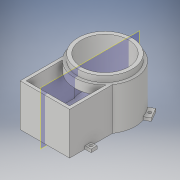
# Autodesk Inventor part: table
Saved by Autodesk Inventor 2018 (Build 220112000, 112)
## iProperties
Created: 2018-04-17
Part Number: table
Material: Generic
Document SubType Name: Modeling
Designer: Cole Tucker
Density: 1 g/cm^3
Appearance: Default
Author: Cole Tucker
Autodesk Inventor part; units mm, degrees
ref_plane "YZ Plane" through (0, 0, 0) normal (1, 0, 0) x (0, 1, 0)
ref_plane "XZ Plane" through (0, 0, 0) normal (0, 1, 0) x (-1, 0, 0)
ref_plane "XY Plane" through (0, 0, 0) normal (0, 0, 1) x (1, 0, 0)
sketch "Sketch1" plane through (0, 0, 0) normal (0, 1, 0) x (-1, 0, 0)
  circle A0 centre (0, 0) radius 24.765
  circle A1 centre (0, 0) radius 28.575
  dimension "d0" = 49.53
  dimension "d1" = 57.15
  constraints: 2 centre point, 2 coincident
  measures "d0" diameter of A0
  measures "d1" diameter of A1
extrude "Extrusion1" add sketch "Sketch1" along normal blind 50.8
sketch "Sketch2" plane through (0, 0, 0) normal (0, -1, 0) x (1, 0, 0)
  circle A0 centre (0, 0) radius 31.75
  circle A1 centre (0, 0) radius 24.765 projected
  circle A2 centre (0, 0) radius 28.575 projected
  circle A3 centre (0, 0) radius 28.575
  dimension "d4" = 63.5
  constraints: 2 centre point, 2 coincident
  measures "d4" diameter of A0
extrude "Extrusion2" add sketch "Sketch2" against normal blind 44.45 contours A0
sketch "Sketch3" plane through (0, 0, 0) normal (0, -1, 0) x (1, 0, 0)
  circle A0 centre (0, 0) radius 24.765 projected
  line L0 (0, 24.765) -> (6.35, 24.765)
  line L1 (6.35, 24.765) -> (6.35, 37.465)
  line L2 (6.35, 37.465) -> (-6.35, 37.465)
  line L3 (-6.35, 37.465) -> (-6.35, 24.765)
  line L4 (-6.35, 24.765) -> (0, 24.765)
  dimension "d7" = 6.35
  dimension "d8" = 12.7
  dimension "d9" = 12.7
  constraints: 10 end point, 3 horizontal, 3 perpendicular, 1 collinear, 1 point on line, 1 vertical alignment, 1 other
  measures "d7" distance of L0.start L0.end
  measures "d8" distance of L0.end L1.end
  measures "d9" distance of L1.end L2.end
extrude "Extrusion3" add sketch "Sketch3" against normal blind 3.175 contours L4 L3 L2 L1 L0
pattern_circular "Circular Pattern3" count 3 over 360 about axis through (0, 0, 0) along (0, 1, 0) of "Extrusion3"
sketch "Sketch5" plane through (0, 3.175, 0) normal (0, 1, 0) x (1, 0, 0)
  line L0 (6.35, -37.465) -> (-6.35, -37.465) projected
  line L1 (0, -37.465) -> (0, -31.75)
  circle A0 centre (0, 0) radius 31.75 projected
  point P0 (0, -34.6075)
  constraints: 2 end point, 2 midpoint, 1 vertical, 1 vertical alignment, 1 other
hole "Hole2" at (0, 3.175, 34.6075) direction (0, -1, 0) diameter 3.175 end through all
pattern_circular "Circular Pattern4" count 3 over 360 about axis through (0, 0, 0) along (0, 1, 0) of "Hole2"
sketch "Sketch6" plane through (-6.35, 0, 37.465) normal (0, 0, 1) x (1, 0, 0)
  line L0 (12.7, 3.175) -> (0, 3.175) projected
  line L1 (6.35, 3.175) -> (6.35, 34.925)
  line L2 (6.35, 34.925) -> (-16.51, 34.925)
  line L3 (-16.51, 34.925) -> (-16.51, 3.175)
  line L4 (-16.51, 3.175) -> (6.35, 3.175)
  line L5 (6.35, 3.175) -> (29.21, 3.175)
  line L6 (29.21, 3.175) -> (29.21, 34.925)
  line L7 (29.21, 34.925) -> (6.35, 34.925)
  point P0 (6.35, 0)
  dimension "d38" = 31.75
  dimension "d39" = 22.86
  dimension "d40" = 22.86
  constraints: 14 end point, 4 perpendicular, 2 point on line, 1 collinear, 1 midpoint, 1 vertical
  measures "d38" distance of L1.start L1.end
  measures "d39" distance of L1.end L2.end
  measures "d40" distance of L1.start L5.end
extrude "Extrusion4" cut sketch "Sketch6" against normal blind 38.1
sketch "Sketch7" plane through (0, 3.175, 0) normal (0, 1, 0) x (1, 0, 0)
  circle A0 centre (0, 0) radius 24.765
  constraints: 1 centre point, 1 coincident
extrude "Extrusion5" add sketch "Sketch7" against normal blind 3.175
sketch "Sketch8" plane through (0, 3.175, 0) normal (0, 1, 0) x (1, 0, 0)
  line L0 (-22.86, -22.0337) -> (-22.86, -9.525) projected
  line L1 (-22.86, -22.0337) -> (22.86, -22.0337)
  line L2 (22.86, -22.0337) -> (22.86, -60.1337)
  line L3 (22.86, -60.1337) -> (-22.86, -60.1337)
  line L4 (-22.86, -60.1337) -> (-22.86, -22.0337)
  point P0 (0, 0)
  dimension "d45" = 38.1
  constraints: 8 end point, 2 parallel, 1 horizontal, 1 perpendicular
  measures "d45" distance of L1.end L2.end
extrude "Extrusion6" add sketch "Sketch8" against normal blind 3.175
sketch "Sketch9" plane through (0, 0, 0) normal (0, -1, 0) x (1, 0, 0)
  line L0 (-22.86, 60.1337) -> (-22.86, 22.0337) projected
  line L1 (-22.86, 60.1337) -> (-26.035, 60.1337)
  line L2 (-26.035, 60.1337) -> (-26.035, 63.3087)
  line L3 (-26.035, 63.3087) -> (-22.86, 63.3087)
  line L4 (-22.86, 63.3087) -> (-22.86, 60.1337)
  line L5 (22.86, 22.0337) -> (22.86, 60.1337) projected
  line L6 (22.86, 60.1337) -> (26.035, 60.1337)
  line L7 (26.035, 60.1337) -> (26.035, 63.3087)
  line L8 (26.035, 63.3087) -> (22.86, 63.3087)
  line L9 (22.86, 63.3087) -> (22.86, 60.1337)
  line L10 (26.035, 60.1337) -> (26.035, 18.1725)
  arc A0 (30.1158, -10.055) -> (22.86, 22.0337) centre (0, 0) ccw projected
  line L11 (-22.86, 63.3087) -> (22.86, 63.3087)
  line L12 (-26.035, 60.1337) -> (-26.035, 18.1725)
  arc A1 (-22.86, 22.0337) -> (-30.1158, -10.055) centre (0, 0) ccw projected
  dimension "d48" = 3.175
  dimension "d49" = 3.175
  dimension "d50" = 3.175
  dimension "d51" = 3.175
  constraints: 22 end point, 4 parallel, 3 perpendicular, 2 horizontal, 2 point on circle, 1 vertical
  measures "d48" distance of L2.end L3.end
  measures "d49" distance of L1.end L2.end
  measures "d50" distance of L8.end L7.end
  measures "d51" distance of L7.end L6.end
extrude "Extrusion7" add sketch "Sketch9" against normal blind 44.45
sketch "Sketch10" plane through (0, 0, 0) normal (0, -1, 0) x (1, 0, 0)
  line L0 (-22.86, 60.1337) -> (-22.86, 63.3087) projected
  line L1 (22.86, 60.1337) -> (-22.86, 60.1337) projected
  line L2 (-22.86, 63.3087) -> (22.86, 63.3087)
  line L3 (22.86, 63.3087) -> (22.86, 60.1337)
  line L4 (22.86, 60.1337) -> (-22.86, 60.1337)
  line L5 (-22.86, 60.1337) -> (-22.86, 63.3087)
  point P0 (0, 0)
  constraints: 8 end point, 2 parallel, 1 horizontal, 1 perpendicular
extrude "Extrusion8" add sketch "Sketch10" against normal blind 44.45
sketch "Sketch11" plane through (0, 0, 0) normal (0, -1, 0) x (1, 0, 0)
  line L0 (-26.035, 18.1725) -> (-26.035, 63.3087) projected
  line L1 (-26.035, 40.7406) -> (-32.385, 40.7406)
  line L2 (-32.385, 40.7406) -> (-32.385, 47.0906)
  line L3 (-32.385, 47.0906) -> (-26.035, 47.0906)
  line L4 (-26.035, 47.0906) -> (-26.035, 40.7406)
  point P0 (0, 0)
  dimension "d56" = 6.35
  dimension "d57" = 6.35
  constraints: 8 end point, 2 parallel, 1 horizontal, 1 midpoint, 1 perpendicular
  measures "d56" distance of L2.end L3.end
  measures "d57" distance of L1.end L2.end
extrude "Extrusion9" add sketch "Sketch11" against normal blind 3.175
sketch "Sketch12" plane through (0, 0, 0) normal (0, -1, 0) x (1, 0, 0)
  line L0 (-26.035, 40.7406) -> (-32.385, 40.7406) projected
  line L1 (-29.21, 40.7406) -> (-29.21, 47.0906)
  line L2 (-32.385, 47.0906) -> (-26.035, 47.0906) projected
  point P0 (0, 0)
  point P1 (-29.21, 43.9156)
  constraints: 3 midpoint, 2 end point
hole "Hole3" at (-29.21, 0, 43.9156) direction (0, 1, 0) diameter 3.175 end through all
ref_plane "Work Plane1" through (0, 0, 63.3087) normal (-1, 0, 0) x (0, 0, 1)
mirror "Mirror1" about plane through (0, 0, 63.3087) normal (-1, 0, 0) of "Extrusion9", "Hole3"
body "Solid1"
